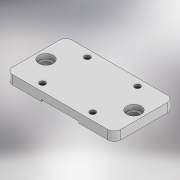
# Autodesk Inventor part: 2021-01-011
Saved by Autodesk Inventor 2020.2 (Build 242310000, 310)
## iProperties
Created: 2021-04-25
Part Number: 2021-01-011
Material: Generic
Document SubType Name: Modeling
Designer: carso
Density: 1 g/cm^3
Appearance: Default
Author: carso
Autodesk Inventor part; units mm, degrees
ref_plane "YZ Plane" through (0, 0, 0) normal (1, 0, 0) x (0, 1, 0)
ref_plane "XZ Plane" through (0, 0, 0) normal (0, 1, 0) x (-1, 0, 0)
ref_plane "Work Plane1" through (0, 0, 0) normal (0, -1, 0) x (1, 0, 0)
sketch "Sketch7" plane through (0, 0, 0) normal (0, 1, 0) x (-1, 0, 0)
  arc A0 (-2, -17) -> (0, -15) centre (-2, -15) ccw
  line L0 (0, -15) -> (0, -2)
  arc A1 (0, -2) -> (-2, 0) centre (-2, -2) ccw
  line L1 (-2, 0) -> (-8.25, 0)
  arc A2 (-6, -2.25) -> (-8.25, 0) centre (-8.25, -2.25) ccw
  line L2 (-6, -14.75) -> (-6, -2.25)
  arc A3 (-8.25, -17) -> (-6, -14.75) centre (-8.25, -14.75) ccw
  line L3 (-8.25, -17) -> (-2, -17)
  line L4 (-22.25, 0) -> (-8.25, 0)
  arc A4 (-22.25, 0) -> (-24.5, -2.25) centre (-22.25, -2.25) ccw
  line L5 (-24.5, -14.75) -> (-24.5, -2.25)
  arc A5 (-24.5, -14.75) -> (-22.25, -17) centre (-22.25, -14.75) ccw
  line L6 (-8.25, -17) -> (-22.25, -17)
  arc A6 (-8.25, -17) -> (-6, -14.75) centre (-8.25, -14.75) ccw
  line L7 (-6, -2.25) -> (-6, -14.75)
  arc A7 (-6, -2.25) -> (-8.25, 0) centre (-8.25, -2.25) ccw
  arc A8 (-28.5, 0) -> (-30.5, -2) centre (-28.5, -2) ccw
  line L8 (-30.5, -2) -> (-30.5, -15)
  arc A9 (-30.5, -15) -> (-28.5, -17) centre (-28.5, -15) ccw
  line L9 (-28.5, -17) -> (-22.25, -17)
  arc A10 (-24.5, -14.75) -> (-22.25, -17) centre (-22.25, -14.75) ccw
  line L10 (-24.5, -2.25) -> (-24.5, -14.75)
  arc A11 (-22.25, 0) -> (-24.5, -2.25) centre (-22.25, -2.25) ccw
  line L11 (-22.25, 0) -> (-28.5, 0)
  line L12 (-23, -4.05) -> (-22.25, -4.05)
  arc A12 (-22.25, -4.05) -> (-20.45, -2.25) centre (-22.25, -2.25) ccw
  line L13 (-20.45, -2.25) -> (-20.45, -1.5)
  arc A13 (-18.95, 0) -> (-20.45, -1.5) centre (-18.95, -1.5) ccw
  line L14 (-18.95, 0) -> (-22.25, 0)
  arc A14 (-22.25, 0) -> (-24.5, -2.25) centre (-22.25, -2.25) ccw
  line L15 (-24.5, -2.25) -> (-24.5, -5.55)
  arc A15 (-23, -4.05) -> (-24.5, -5.55) centre (-23, -5.55) ccw
  circle A16 centre (-22.25, -2.25) radius 0.8
  line L16 (-8.25, -4.05) -> (-7.5, -4.05)
  arc A17 (-6, -5.55) -> (-7.5, -4.05) centre (-7.5, -5.55) ccw
  line L17 (-6, -5.55) -> (-6, -2.25)
  arc A18 (-6, -2.25) -> (-8.25, 0) centre (-8.25, -2.25) ccw
  line L18 (-8.25, 0) -> (-11.55, 0)
  arc A19 (-10.05, -1.5) -> (-11.55, 0) centre (-11.55, -1.5) ccw
  line L19 (-10.05, -1.5) -> (-10.05, -2.25)
  arc A20 (-10.05, -2.25) -> (-8.25, -4.05) centre (-8.25, -2.25) ccw
  circle A21 centre (-8.25, -2.25) radius 0.8
  line L20 (-10.05, -14.75) -> (-10.05, -15.5)
  arc A22 (-11.55, -17) -> (-10.05, -15.5) centre (-11.55, -15.5) ccw
  line L21 (-11.55, -17) -> (-8.25, -17)
  arc A23 (-8.25, -17) -> (-6, -14.75) centre (-8.25, -14.75) ccw
  line L22 (-6, -14.75) -> (-6, -11.45)
  arc A24 (-7.5, -12.95) -> (-6, -11.45) centre (-7.5, -11.45) ccw
  line L23 (-7.5, -12.95) -> (-8.25, -12.95)
  arc A25 (-8.25, -12.95) -> (-10.05, -14.75) centre (-8.25, -14.75) ccw
  circle A26 centre (-8.25, -14.75) radius 0.8
  line L24 (-22.25, -12.95) -> (-23, -12.95)
  arc A27 (-24.5, -11.45) -> (-23, -12.95) centre (-23, -11.45) ccw
  line L25 (-24.5, -11.45) -> (-24.5, -14.75)
  arc A28 (-24.5, -14.75) -> (-22.25, -17) centre (-22.25, -14.75) ccw
  line L26 (-22.25, -17) -> (-18.95, -17)
  arc A29 (-20.45, -15.5) -> (-18.95, -17) centre (-18.95, -15.5) ccw
  line L27 (-20.45, -15.5) -> (-20.45, -14.75)
  arc A30 (-20.45, -14.75) -> (-22.25, -12.95) centre (-22.25, -14.75) ccw
  circle A31 centre (-22.25, -14.75) radius 0.8
  line L28 (-10.05, -1.5) -> (-10.05, 0)
  line L29 (-10.05, -15.5) -> (-10.05, -17)
  line L30 (-20.45, -15.5) -> (-20.45, -17)
  line L31 (-20.45, -1.5) -> (-20.45, 0)
  point P0 (0, 0)
  point P1 (145.09, 90.0262)
  point P2 (-71.3045, 9.3)
  point P3 (-8.25, 0)
  point P4 (-6, -5.55)
  constraints: 64 end point, 56 point on circle, 32 centre point, 6 point on line, 2 perpendicular, 2 tangent
extrude "Extrusion5" add sketch "Sketch7" along normal blind 2.52 contours L3 A3 L2 A2 L1 A1 L0 A0 | L6 L29 L20 A25 L23 A24 L2 A3 | L6 A22 L29 | A24 L23 A25 L20 A22 L6 A29 L27 A30 L24 A27 L5 A15 L12 A12 L13 A13 L4 A19 L19 A20 L16 A17 L2 | A2 L2 A17 L16 A20 L19 L28 L4 | L6 L30 A29 | L28 A19 L4 | L6 A5 L5 A27 L24 A30 L27 L30 | L9 A9 L8 A8 L11 A4 L5 A5 | A13 L31 L4 | L31 L13 A12 L12 A15 L5 A4 L4 | A16 | A21 | A26 | A31
extrude "Extrusion6" cut sketch "Sketch7" along normal blind 0.5 contours L6 A22 L29 | A24 L23 A25 L20 A22 L6 A29 L27 A30 L24 A27 L5 A15 L12 A12 L13 A13 L4 A19 L19 A20 L16 A17 L2 | L6 L30 A29 | L28 A19 L4 | A13 L31 L4
sketch "Sketch8" plane through (0, 2.52, 0) normal (0, 1, 0) x (1, 0, 0)
  arc A0 (0, 2) -> (2, 0) centre (2, 2) ccw projected
  line L0 (2, 0) -> (28.5, 0) projected
  arc A1 (28.5, 0) -> (30.5, 2) centre (28.5, 2) ccw projected
  line L1 (30.5, 2) -> (30.5, 15) projected
  arc A2 (30.5, 15) -> (28.5, 17) centre (28.5, 15) ccw projected
  line L2 (28.5, 17) -> (2, 17) projected
  arc A3 (2, 17) -> (0, 15) centre (2, 15) ccw projected
  line L3 (0, 15) -> (0, 2) projected
  line L4 (2, 16.8) -> (28.5, 16.8)
  arc A4 (30.3, 15) -> (28.5, 16.8) centre (28.5, 15) ccw
  line L5 (30.3, 15) -> (30.3, 2)
  arc A5 (28.5, 0.2) -> (30.3, 2) centre (28.5, 2) ccw
  line L6 (28.5, 0.2) -> (2, 0.2)
  arc A6 (0.2, 2) -> (2, 0.2) centre (2, 2) ccw
  line L7 (0.2, 2) -> (0.2, 15)
  arc A7 (2, 16.8) -> (0.2, 15) centre (2, 15) ccw
  point P0 (0, 0)
  dimension "d32" = 0.2
  constraints: 8 end point, 8 point on circle, 4 centre point, 7 other
  measures "d32" distance between parallel lines of L2 L4
extrude "Extrusion7" cut sketch "Sketch8" against normal blind 10
hole "Hole3" at (22.25, 0, -14.75) at (8.25, 0, -14.75) at (8.25, 0, -2.25) at (22.25, 0, -2.25) direction (0, 1, 0) diameter 1.567 depth 3 thread size "M2x0.4" class "6H" standard "ISO Metric profile"
sketch "Sketch10" plane through (0, 2.52, 0) normal (0, 1, 0) x (1, 0, 0)
  line L0 (24.5, 14.75) -> (24.5, 2.25) projected
  line L1 (6, 14.75) -> (6, 2.25) projected
  line L2 (24.5, 5.55) -> (24.5, 11.45) projected
  line L3 (24.5, 8.5) -> (27.5, 8.5)
  line L4 (6, 11.45) -> (6, 5.55) projected
  line L5 (6, 8.5) -> (3, 8.5)
  point P0 (0, 0)
  dimension "d42" = 3
  dimension "d43" = 3
  constraints: 4 end point, 2 horizontal, 2 midpoint
  measures "d42" distance of L3.start L3.end
  measures "d43" distance of L5.start L5.end
hole "Hole4" at (27.5, 2.52, -8.5) at (3, 2.52, -8.5) direction (0, -1, 0) diameter 2.4 depth 3 counterbore diameter 4 counterbore depth 1.35
body "Solid2"
